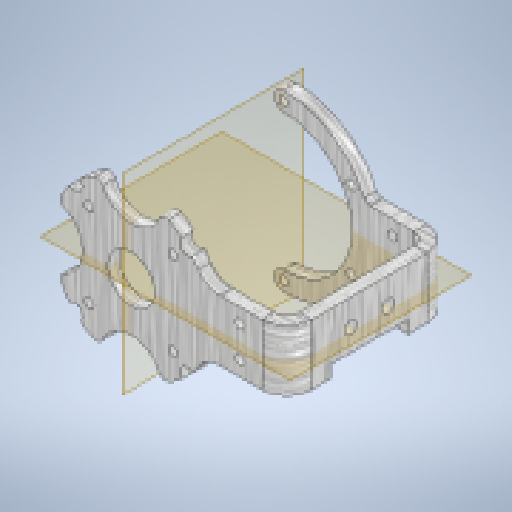
# Autodesk Inventor part: J3_J4_CONNECTOR
Saved by Autodesk Inventor 2025.4 (Build 294407000, 407)
## iProperties
Created: 2026-06-27
Part Number: J3_J4_CONNECTOR
Material: 铝 5052
Document SubType Name: 钣金
Designer: Admin
Density: 2.68 g/cm^3
Appearance: 缎光 - 强拉丝
Sheet Metal Rule: 默认
Author: Admin
Autodesk Inventor part; units mm, degrees
ref_plane "XY Plane" through (0, 0, 0) normal (0, 0, 1) x (1, 0, 0)
sketch "草图2" plane through (0, 0, 0) normal (0, 0, 1) x (1, 0, 0)
  circle A0 centre (-18.0312, 18.0312) radius 2.5
  circle A1 centre (-13.435, 13.435) radius 1.35
  circle A2 centre (0, 0) radius 25.5
  circle A3 centre (-13.435, 13.435) radius 1.5
  circle A4 centre (-13.435, -13.435) radius 1.5
  circle A5 centre (-18.0312, -18.0312) radius 2.5
  circle A6 centre (13.435, -13.435) radius 1.5
  circle A7 centre (18.0312, -18.0312) radius 2.5
  circle A8 centre (13.435, 13.435) radius 1.5
  circle A9 centre (18.0312, 18.0312) radius 2.5
  circle A10 centre (0, -25.5) radius 10
  line L0 (0, 49.7) -> (0, -49.7) projected
  line L1 (-54.2911, 0) -> (77.2468, 0) projected
  circle A11 centre (-25.5, 0) radius 10
  circle A12 centre (0, 25.5) radius 10
  line L2 (35, -9.75) -> (35, 9.75)
  line L3 (35, -9.75) -> (28.411, -9.75)
  line L4 (28.411, -9.75) -> (28.411, 9.75)
  line L5 (28.411, 9.75) -> (35, 9.75)
  line L6 (35, 9.75) -> (35, -9.75)
  arc A13 (28.411, -9.75) -> (21.6263, -13.5112) centre (28.411, -17.75) ccw
  arc A14 (21.6263, 13.5112) -> (28.411, 9.75) centre (28.411, 17.75) ccw
  line L7 (21.6263, -13.5112) -> (21.6263, 13.5112)
  circle A15 centre (0, 0) radius 7.5
  point P0 (46.5273, 9.0663)
  point P1 (58.4557, 0)
  point P2 (-26.1005, -20)
  point P3 (35, 0)
  point P4 (9.8059, -23.5392)
  point P5 (16.1789, -19.7102)
  point P6 (19.7102, -16.1789)
  point P7 (19.7102, 16.1789)
  point P8 (16.1789, 19.7102)
  point P9 (9.8059, 23.5392)
  point P10 (-9.8059, 23.5392)
  point P11 (-16.1789, 19.7102)
  point P12 (-19.7102, 16.1789)
  point P13 (-23.5392, 9.8059)
  point P14 (-23.5392, -9.8059)
  point P15 (-19.7102, -16.1789)
  point P16 (-16.1789, -19.7102)
  point P17 (-9.8059, -23.5392)
  dimension "d171" = 3
  dimension "d174" = 360
  dimension "d176" = 20
  dimension "d177" = 20
  dimension "d178" = 20
  dimension "d179" = 19.5
  dimension "d181" = 35
  dimension "d182" = 8
  dimension "d183" = 15
  constraints: 16 centre point, 12 end point, 10 point on circle, 5 point on line, 4 tangent, 3 parallel, 2 coincident, 2 midpoint, 2 perpendicular, 1 equal radius, 1 horizontal, 22 other
  measures "d171" diameter of A3
  measures "d176" diameter of A10
  measures "d177" diameter of A11
  measures "d178" diameter of A12
  measures "d179" distance of L2.start L2.end
  measures "d181" distance from line of A2.centre L2
  measures "d182" radius of A14
  measures "d183" diameter of A15
extrude "拉伸1" add sketch "草图2" along normal blind 4 contours A0 A2 A12 L0 A15 L1 A11 | A12 A2 A9 L7 L1 A15 L0 | L1 A15 L0 A10 A2 A5 A11 | L1 L7 A2 A7 A10 L0 A15 | L7 A2 L1 | L1 A2 L7 | A14 L4 L1 A2 | L1 L4 A13 A2 | L5 L2 L1 L4 | L1 L2 L3 L4
sketch "草图15" plane through (35, -9.75, 0) normal (1, 0, 0) x (0, 0, -1)
  line L0 (0, 0) -> (0, 19.5) projected
  line L1 (0, 19.5) -> (-4, 19.5) projected
  line L2 (-4, 0) -> (-4, 19.5) projected
  line L3 (0, 0) -> (-4, 0) projected
  point P0 (0, 9.75)
extrude "拉伸10" add sketch "草图15" along normal blind 11
sketch "草图17" plane through (46, -9.75, 0) normal (1, 0, 0) x (0, 1, 0)
  line L0 (19.5, 0) -> (0, 0)
  line L1 (0, 0) -> (0, -45)
  line L2 (0, -45) -> (19.5, -45)
  line L3 (19.5, -45) -> (19.5, 0)
  constraints: 6 end point, 1 horizontal, 1 perpendicular, 1 vertical
edge flange "凸缘4" height 45 angle 90 thickness 4 bend radius 4 thickness toward (1, 0, 0) relief tear relief width 4 relief depth 2 edges at (46, 0, 0) wall of the first edge with corners at (46, 9.75, 0) (46, -9.75, 0) (46, -9.75, -45) (46, 9.75, -45)
bend "折弯4"
corner "拐角4"
sketch "草图18" plane through (46, -9.75, -45) normal (0, 0, -1) x (-1, 0, 0)
  line L0 (0, 19.5) -> (0, 0)
  line L1 (0, 0) -> (20, 0)
  line L2 (20, 0) -> (20, 19.5)
  line L3 (20, 19.5) -> (0, 19.5)
  constraints: 6 end point, 1 horizontal, 1 perpendicular, 1 vertical
edge flange "凸缘5" height 20 angle 90 thickness 4 bend radius 4 thickness toward (0, 0, -1) relief tear relief width 4 relief depth 2 edges at (46, 0, -45) wall of the first edge with corners at (46, 9.75, -45) (46, -9.75, -45) (26, -9.75, -45) (26, 9.75, -45)
bend "折弯5"
corner "拐角5"
sketch "草图22" plane through (26, -9.75, -49) normal (0, 0, -1) x (-1, 0, 0)
  circle A0 centre (26, -15.25) radius 1.25
  circle A1 centre (4.3494, -2.75) radius 1.25
  circle A2 centre (4.3494, 22.25) radius 1.35
  circle A3 centre (26, 34.75) radius 1.25
  circle A4 centre (26, 34.75) radius 3
  circle A5 centre (26, 34.75) radius 1.5
  circle A6 centre (4.3494, 22.25) radius 1.5
  circle A7 centre (4.3494, -2.75) radius 1.5
  circle A8 centre (26, -15.25) radius 1.5
  circle A9 centre (26, -15.25) radius 3
  circle A10 centre (26, 9.75) radius 7.5
  arc A11 (26, 31.75) -> (26, -12.25) centre (26, 9.75) ccw
  arc A12 (16.1941, 33.2892) -> (9.8211, 29.4602) centre (26, 9.75) ccw
  arc A13 (26, 37.75) -> (26, -18.25) centre (26, 9.75) ccw
  dimension "d184" = 6
  dimension "d185" = 3
  dimension "d186" = 3
  dimension "d187" = 3
  dimension "d188" = 3
  dimension "d189" = 6
  measures "d184" diameter of A4
  measures "d185" diameter of A5
  measures "d186" diameter of A6
  measures "d187" diameter of A7
  measures "d188" diameter of A8
  measures "d189" diameter of A9
sheet face with bend "平板1" sketch "草图22" thickness 4 toward (0, 0, 1) bend radius 4 contours A4 | A4 A11 A9 A13 | A9
bend "折弯6"
sketch "草图23" plane through (50, -9.75, -4) normal (1, 0, 0) x (0, 0, -1)
  line L0 (37, 0) -> (0, 0) projected
  line L1 (31, 0) -> (6, 0)
  line L2 (6, 0) -> (6, 4)
  line L3 (6, 4) -> (31, 4)
  line L4 (31, 4) -> (31, 0)
  point P0 (-4, 9.75)
  point P1 (18.5, 0)
  point P2 (18.5, 4)
  point P3 (18.5, 0)
  point P4 (6, 0)
  dimension "d153" = 25
  dimension "d154" = 4
  constraints: 8 end point, 3 midpoint, 2 parallel, 1 coincident, 1 horizontal, 1 perpendicular, 1 point on line, 1 vertical alignment
  measures "d153" distance of L2.end L3.end
  measures "d154" distance of L3.end L1.start
extrude "拉伸11" cut sketch "草图23" against normal blind 10
sketch "草图24" plane through (50, -9.75, -4) normal (1, 0, 0) x (0, 0, -1)
  circle A0 centre (24.5, 11) radius 2
  circle A1 centre (12.5, 11) radius 2
  line L0 (24.5, 11) -> (12.5, 11)
  line L1 (6, 4) -> (31, 4) projected
  line L2 (37, 0) -> (37, 19.5) projected
  point P0 (-4, 9.75)
  point P1 (18.5, 11)
  point P2 (18.5, 4)
  point P3 (37, 9.75)
  dimension "d157" = 4
  dimension "d158" = 7
  dimension "d159" = 12
  constraints: 3 midpoint, 2 centre point, 2 end point, 1 vertical alignment
  measures "d157" diameter of A0
  measures "d158" distance between parallel lines of L1 L0
  measures "d159" distance of L0.start L0.end
extrude "拉伸12" cut sketch "草图24" against normal blind 10
sketch "草图25" plane through (0, 0, 4) normal (0, 0, 1) x (1, 0, 0)
  line L0 (42, -9.75) -> (42, 9.75) projected
  line L1 (33, -5) -> (33, 5)
  line L2 (0, 39.2) -> (0, -39.2) projected
  point P0 (0, 0)
  point P1 (33, 0)
  dimension "d163" = 10
  dimension "d192" = 33
  constraints: 2 end point, 1 horizontal alignment, 1 midpoint, 1 vertical, 1 vertical alignment
  measures "d163" distance of L1.start L1.end
  measures "d192" distance between parallel lines of L2 L1
hole "孔2" at (33, -5, 4) at (33, 5, 4) direction (0, 0, -1) diameter 3 end through all
fillet "圆角3" radius 2 6 edges at (-23.5392, -9.8059, 2) (-23.5392, 9.8059, 2) (9.8059, 23.5392, 2) (9.8059, -23.5392, 2) (-9.8059, -23.5392, 2) (-9.8059, 23.5392, 2)
fillet "圆角4" radius 2 2 edges at (26.2476, 9.75, -47) (26.2476, -9.75, -47)
